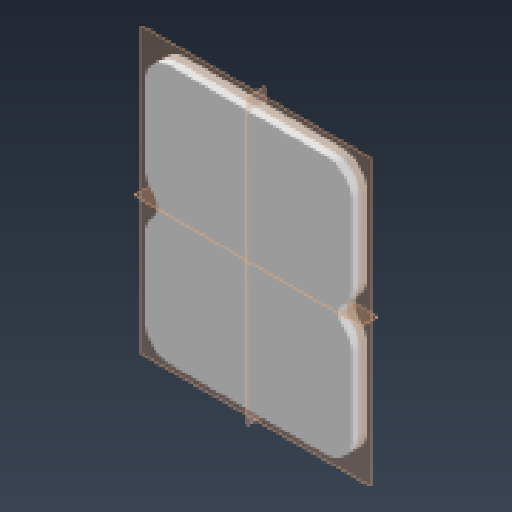
# Autodesk Inventor part: Фанерка_маркера
Saved by Autodesk Inventor 2023.2 (Build 272271030, 271C)
## iProperties
Created: 2026-01-04
Part Number: Фанерка_маркера
Material: Типовые
Document SubType Name: Modeling
Designer: Олег Коноваленко
Density: 1 g/cm^3
Appearance: По умолчанию
Author: Олег Коноваленко
Autodesk Inventor part; units mm, degrees
sketch "Эскиз1" plane through (0, 0, 0) normal (0, 0, 1) x (1, 0, 0)
  line L0 (-20, 25) -> (20, 25)
  line L1 (20, 25) -> (20, -25)
  line L2 (20, -25) -> (-20, -25)
  line L3 (-20, -25) -> (-20, 25)
  line L4 (-20, 25) -> (20, -25) construction
  line L5 (20, 25) -> (-20, -25) construction
  point P0 (0, 0)
  dimension "d0" = 50
  dimension "d1" = 40
  constraints: 12 end point, 2 midpoint, 2 parallel, 1 horizontal, 1 perpendicular
  measures "d0" distance of L0.end L1.end
  measures "d1" distance of L1.end L2.end
extrude "Выдавливание1" add sketch "Эскиз1" along normal mid plane 3
fillet "Сопряжение1" radius 5 4 edges at (20, -25, 0) (20, 25, 0) (-20, 25, 0) (-20, -25, 0)
sketch "Эскиз2" plane through (0, 0, -1.5) normal (0, 0, -1) x (-1, 0, 0)
  line L0 (-20, -20) -> (-20, 20) projected
  circle A0 centre (-20, 0) radius 2.5
  line L1 (20, -20) -> (20, 20) projected
  circle A1 centre (20, 0) radius 2.5
  point P0 (0, 0)
  point P1 (20, 2.5)
  point P2 (20, -2.5)
  point P3 (-20, 2.5)
  point P4 (-20, -2.5)
  dimension "d5" = 5
  constraints: 2 centre point, 2 midpoint, 1 equal radius
  measures "d5" diameter of A0
extrude "Выдавливание2" cut sketch "Эскиз2" against normal up to next contours L0 A0 | A1 L1 picked at (-19.4804, 0.6515) picked at (19.1727, 0.1004)
fillet "Сопряжение2" radius 5 4 edges at (-20, 2.5, 0) (-20, -2.5, 0) (20, -2.5, 0) (20, 2.5, 0)
